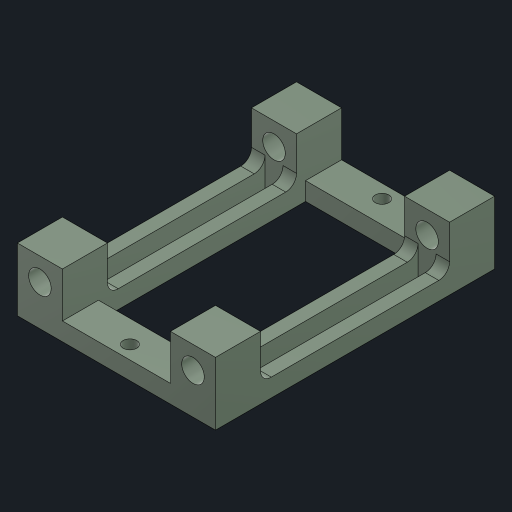
# Autodesk Inventor part: om_DropBase_8g
Saved by Autodesk Inventor 2023 (Build 270158000, 158)
## iProperties
Created: 2022-06-07
Part Number: om_DropBase_8g
Material: ABS プラスチック
Document SubType Name: Modeling
Designer: legot
Density: 1.06 g/cm^3
Appearance: 滑らか - 白
Author: legot
Autodesk Inventor part; units mm, degrees
ref_plane "YZ Plane" through (0, 0, 0) normal (1, 0, 0) x (0, 1, 0)
ref_plane "XZ Plane" through (0, 0, 0) normal (0, 1, 0) x (-1, 0, 0)
ref_plane "XY Plane" through (0, 0, 0) normal (0, 0, 1) x (1, 0, 0)
sketch "スケッチ1" plane through (0, 0, 0) normal (0, 1, 0) x (-1, 0, 0)
  line L0 (6, 11.5) -> (-6, 11.5)
  line L1 (-6, 11.5) -> (-6, -11.5)
  line L2 (-6, -11.5) -> (6, -11.5)
  line L3 (6, -11.5) -> (6, 11.5)
  line L4 (6, -11.5) -> (-6, 11.5) construction
  line L5 (6, 11.5) -> (-6, -11.5) construction
  line L6 (11, 11.5) -> (11, -11.5)
  line L7 (-11, 11.5) -> (-11, -11.5)
  line L8 (0, 4) -> (0, -4) construction
  line L9 (0, 14) -> (0, -14) construction
  line L10 (11, -11.5) -> (11, -15.5)
  line L11 (11, -15.5) -> (-11, -15.5)
  line L12 (-11, -15.5) -> (-11, -11.5)
  line L13 (-11, 11.5) -> (-11, 15.5)
  line L14 (-11, 15.5) -> (11, 15.5)
  line L15 (11, 15.5) -> (11, 11.5)
  point P0 (0, 0)
  point P1 (0, 0)
  point P2 (0, 0)
  point P3 (0, -14)
  dimension "d0" = 23
  dimension "d1" = 12
  dimension "d2" = 5
  dimension "d3" = 28
  dimension "d4" = 8
  dimension "d21" = 4
  dimension "d26" = 5
  dimension "d27" = 4
  constraints: 32 end point, 6 midpoint, 6 vertical, 5 perpendicular, 4 coincident, 4 parallel, 2 horizontal alignment, 1 horizontal
  measures "d0" distance of L2.end L0.start
  measures "d1" distance of L1.end L2.end
  measures "d2" distance between parallel lines of L6 L3
  measures "d3" distance of L9.start L9.end
  measures "d4" distance of L8.start L8.end
  measures "d21" distance between parallel lines of L11 L2
  measures "d26" distance between parallel lines of L7 L1
  measures "d27" distance between parallel lines of L14 L0
extrude "押し出し1" add sketch "スケッチ1" along normal blind 2
hole "穴1" at (0, 0, 4) at (0, 0, -4) at (0, 0, 14) at (0, 0, -14) direction (0, 1, 0) diameter 1.5 end through all
sketch "スケッチ2" plane through (0, 2, 0) normal (0, 1, 0) x (1, 0, 0)
  line L0 (-6, -11.5) -> (-6, 11.5) projected
  circle A0 centre (0, -14) radius 0.75 projected
  circle A1 centre (0, 14) radius 0.75 projected
  line L1 (-11, 15.5) -> (-11, -15.5) projected
  line L2 (11, -15.5) -> (11, 15.5) projected
  line L3 (11, 15.5) -> (-11, 15.5) projected
  line L4 (-11, -15.5) -> (11, -15.5) projected
  line L5 (-11, 15.5) -> (-11, -15.5) projected
  line L6 (-11, -15.5) -> (11, -15.5) projected
  line L7 (-6, -15.5) -> (-11, -15.5)
  line L8 (-11, -15.5) -> (-11, -10.5)
  line L9 (-11, -10.5) -> (-6, -10.5)
  line L10 (-6, -10.5) -> (-6, -15.5)
  line L11 (6, -11.5) -> (-6, -11.5) projected
  line L12 (-6, -11.5) -> (-6, 11.5) projected
  line L13 (-6, 11.5) -> (6, 11.5) projected
  line L14 (6, 11.5) -> (6, -11.5) projected
  point P0 (0, 0)
  point P1 (-6, -10.5)
  dimension "d28" = 5
  constraints: 8 end point, 2 parallel, 2 point on line, 1 collinear, 1 horizontal, 1 perpendicular
  measures "d28" distance of L9.end L7.start
extrude "押し出し2" add sketch "スケッチ2" along normal blind 5 contours L10 L4 L1 L9 L0
sketch "スケッチ6" plane through (-6, 2, 10.5) normal (0, 0, -1) x (-1, 0, 0)
  line L0 (5, 0) -> (0, 5) construction
  line L1 (5, 5) -> (0, 0) construction
  circle A0 centre (2.5, 2.5) radius 1.25
  point P0 (-6, -2)
  dimension "d29" = 2.5
  constraints: 4 end point, 1 centre point, 1 midpoint
  measures "d29" diameter of A0
extrude "押し出し5" cut sketch "スケッチ6" along normal through all both and the other way through all
mirror "ミラー4" about plane through (0, 0, 0) normal (0, 0, 1) of "押し出し2", "押し出し5"
sketch "スケッチ7" plane through (0, 2, 0) normal (0, 1, 0) x (1, 0, 0)
  line L0 (-6, 10.5) -> (-11, 10.5) projected
  line L1 (-11, -10.5) -> (-6, -10.5) projected
  line L2 (-6, -10.5) -> (-11, 10.5) construction
  line L3 (-6, 10.5) -> (-11, -10.5) construction
  line L4 (-7.5, -10.5) -> (-9.5, -10.5)
  line L5 (-9.5, -10.5) -> (-9.5, 10.5)
  line L6 (-9.5, 10.5) -> (-7.5, 10.5)
  line L7 (-7.5, 10.5) -> (-7.5, -10.5)
  line L8 (-7.5, -10.5) -> (-9.5, 10.5) construction
  point P0 (0, 0)
  point P1 (-8.5, 0)
  dimension "d32" = 2
  constraints: 14 end point, 3 midpoint, 2 parallel, 1 collinear, 1 horizontal, 1 perpendicular
  measures "d32" distance between parallel lines of L7 L5
extrude "押し出し6" cut sketch "スケッチ7" against normal through all
mirror "ミラー5" about plane through (0, 0, 0) normal (1, 0, 0) of "押し出し2", "押し出し5", "ミラー4", "押し出し6"
fillet "フィレット1" radius 1.2 8 edges at (-10.25, 2, -10.5) (-6.75, 2, -10.5) (6.75, 2, -10.5) (10.25, 2, -10.5) (-10.25, 2, 10.5) (-6.75, 2, 10.5) (6.75, 2, 10.5) (10.25, 2, 10.5)
ref_plane "作業平面1" through (8.5, 0, 15.5) normal (1, 0, 0) x (0, 0, -1)
ref_plane "作業平面2" through (-8.5, 0, 11.5) normal (1, 0, 0) x (0, 0, -1)
equation "\"d26\" = d2"
equation "\"d27\" = d21"
